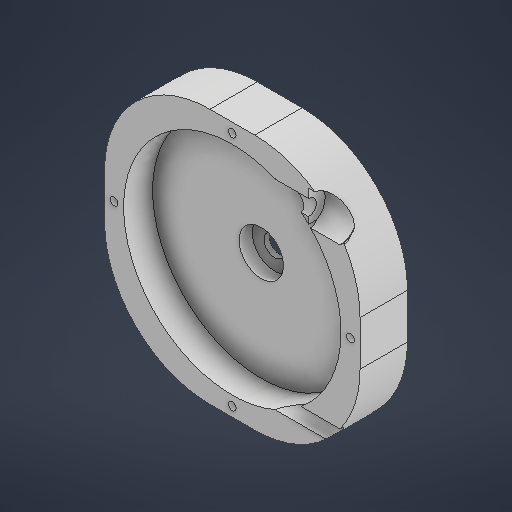
# Autodesk Inventor part: Case
Saved by Autodesk Inventor 2025.3 (Build 293356030, 356C)
## iProperties
Created: 2025-10-02
Part Number: Case
Material: Generic
Document SubType Name: Modeling
Designer: yo
Density: 1 g/cm^3
Appearance: Default
Author: yo
Autodesk Inventor part; units mm, degrees
ref_plane "YZ Plane" through (0, 0, 0) normal (1, 0, 0) x (0, 1, 0)
ref_plane "XZ Plane" through (0, 0, 0) normal (0, 1, 0) x (-1, 0, 0)
ref_plane "XY Plane" through (0, 0, 0) normal (0, 0, 1) x (1, 0, 0)
sketch "Sketch1" plane through (0, 0, 0) normal (0, 0, 1) x (1, 0, 0)
  line L0 (-8.5, 48.5) -> (8.5, 48.5)
  line L1 (48.5, 8.5) -> (48.5, -8.5)
  line L2 (8.5, -48.5) -> (-8.5, -48.5)
  line L3 (-48.5, -8.5) -> (-48.5, 8.5)
  circle A0 centre (0, 0) radius 41.25
  circle A1 centre (0, 0) radius 8.45
  circle A2 centre (0, 0) radius 4
  arc A3 (48.5, 8.5) -> (8.5, 48.5) centre (8.5, 8.5) ccw
  arc A4 (8.5, -48.5) -> (48.5, -8.5) centre (8.5, -8.5) ccw
  arc A5 (-48.5, -8.5) -> (-8.5, -48.5) centre (-8.5, -8.5) ccw
  arc A6 (-8.5, 48.5) -> (-48.5, 8.5) centre (-8.5, 8.5) ccw
  point P0 (-48.5, 48.5)
  point P1 (48.5, -48.5)
  point P2 (48.5, 48.5)
  point P3 (-48.5, -48.5)
  point P4 (0, 48.5)
  point P5 (48.5, 0)
  dimension "d0" = 97
  dimension "d1" = 82.5
  dimension "d2" = 16.9
  dimension "d3" = 8
  dimension "d10" = 40
  constraints: 8 end point, 8 point on circle, 8 point on line, 8 tangent, 7 centre point, 3 coincident, 3 equal radius, 2 midpoint, 2 parallel, 2 perpendicular, 1 horizontal, 1 horizontal alignment, 1 vertical alignment
  measures "d0" distance of point (-48.5, 48.5) point (48.5, 48.5)
  measures "d1" diameter of A0
  measures "d2" diameter of A1
  measures "d3" diameter of A2
  measures "d10" radius of A3
extrude "Extrusion1" add sketch "Sketch1" along normal blind 2 contours A1
extrude "Extrusion2" add sketch "Sketch1" along normal blind 7 contours A0
extrude "Extrusion3" add sketch "Sketch1" along normal blind 18 contours L0 A3 L1 A4 L2 A5 L3 A6
sketch "Sketch3" plane through (0, 0, 18) normal (0, 0, 1) x (1, 0, 0)
  circle A0 centre (0, 0) radius 41.25
  line L0 (21.9501, 34.925) -> (64.9501, 34.925)
  line L1 (41.9501, 40.25) -> (47.9501, 40.25)
  line L2 (49.9501, 42.25) -> (64.9501, 42.25)
  line L3 (40.9501, 41.25) -> (28.9501, 41.25)
  line L4 (49.9501, 42.25) -> (47.9501, 40.25)
  line L5 (40.9501, 41.25) -> (41.9501, 40.25)
  line L6 (47.9501, 40.25) -> (64.9501, 40.25) construction
  line L7 (41.9501, 40.25) -> (28.9501, 40.25) construction
  line L8 (64.9501, 42.25) -> (64.9501, 34.925)
  line L9 (28.9501, 37.925) -> (21.9501, 37.925)
  line L10 (28.9501, 37.925) -> (28.9501, 41.25)
  line L11 (21.9501, 37.925) -> (21.9501, 34.925) construction
  line L12 (21.9501, 34.925) -> (16.225193, 34.925)
  line L13 (21.9501, 37.925) -> (16.225193, 37.925)
  line L14 (16.225193, 34.925) -> (16.225193, 37.925)
  circle A1 centre (0, 0) radius 4
  line L15 (0, 0) -> (48.5, 0)
  line L16 (48.5, -8.5) -> (48.5, 8.5)
  line L17 (21.9501, -34.925) -> (64.9501, -34.925)
  line L18 (41.9501, -40.25) -> (47.9501, -40.25)
  line L19 (49.9501, -42.25) -> (64.9501, -42.25)
  line L20 (40.9501, -41.25) -> (28.9501, -41.25)
  line L21 (49.9501, -42.25) -> (47.9501, -40.25)
  line L22 (40.9501, -41.25) -> (41.9501, -40.25)
  line L23 (47.9501, -40.25) -> (64.9501, -40.25) construction
  line L24 (41.9501, -40.25) -> (28.9501, -40.25) construction
  line L25 (64.9501, -42.25) -> (64.9501, -34.925)
  line L26 (28.9501, -37.925) -> (21.9501, -37.925)
  line L27 (28.9501, -37.925) -> (28.9501, -41.25)
  line L28 (21.9501, -37.925) -> (21.9501, -34.925) construction
  line L29 (21.9501, -34.925) -> (16.225193, -34.925)
  line L30 (21.9501, -37.925) -> (16.225193, -37.925)
  line L31 (16.225193, -34.925) -> (16.225193, -37.925)
  line L32 (28.9501, -37.925) -> (64.9501, -37.925)
  point P0 (16.225193, -37.925)
  dimension "d12" = 10.65
  dimension "d13" = 14.65
  dimension "d14" = 12.65
  dimension "d15" = 45
  dimension "d16" = 45
  dimension "d17" = 15
  dimension "d18" = 6
  dimension "d19" = 12
  dimension "d21" = 7
  dimension "d22" = 6
  constraints: 64 end point, 14 symmetric about line, 9 horizontal, 4 vertical, 4 vertical alignment, 2 point on circle, 1 midpoint, 1 perpendicular, 1 point on line, 1 tangent
  measures "d12" diameter of L1 L0
  measures "d13" diameter of L2 L0
  measures "d14" diameter of L3 L0
  measures "d15" angle of L6 L4
  measures "d16" angle of L5 L7
  measures "d17" distance of L2.start L2.end
  measures "d18" distance of L1.start L1.end
  measures "d19" distance of L3.start L3.end
  measures "d21" distance of L9.start L9.end
  measures "d22" diameter of L9 L0
sketch "Sketch3 outline for Revolution1" plane through (0, 0, 18) normal (0, 0, 1) x (1, 0, 0)
  line L0 (64.9501, 34.925) -> (64.9501, 42.25)
  line L1 (21.9501, 34.925) -> (64.9501, 34.925)
  arc A0 (16.225193, 37.925) -> (21.9501, 34.925) centre (0, 0) cw
  line L2 (21.9501, 37.925) -> (16.225193, 37.925)
  line L3 (28.9501, 37.925) -> (21.9501, 37.925)
  line L4 (28.9501, 41.25) -> (28.9501, 37.925)
  line L5 (40.9501, 41.25) -> (28.9501, 41.25)
  line L6 (41.9501, 40.25) -> (40.9501, 41.25)
  line L7 (47.9501, 40.25) -> (41.9501, 40.25)
  line L8 (49.9501, 42.25) -> (47.9501, 40.25)
  line L9 (64.9501, 42.25) -> (49.9501, 42.25)
revolve "Revolution1" cut sketch "Sketch3 outline for Revolution1" angle 360 about axis through (21.9501, 34.925, 18) along (1, 0, 0)
sketch "Sketch3 outline for Revolution2" plane through (0, 0, 18) normal (0, 0, 1) x (1, 0, 0)
  line L0 (21.9501, -37.925) -> (28.9501, -37.925)
  line L1 (16.225193, -37.925) -> (21.9501, -37.925)
  arc A0 (21.9501, -34.925) -> (16.225193, -37.925) centre (0, 0) cw
  line L2 (64.9501, -34.925) -> (21.9501, -34.925)
  line L3 (64.9501, -37.925) -> (64.9501, -34.925)
  line L4 (28.9501, -37.925) -> (64.9501, -37.925)
revolve "Revolution2" cut sketch "Sketch3 outline for Revolution2" angle 360 about axis through (21.9501, -34.925, 18) along (1, 0, 0)
sketch "Sketch4" plane through (0, 0, 18) normal (0, 0, 1) x (1, 0, 0)
  line L0 (35.59556, -37.925) -> (16.225193, -37.925) construction
  arc A0 (16.225193, 37.925) -> (16.225193, -37.925) centre (0, 0) ccw construction
  line L1 (16.225193, 37.925) -> (28.9501, 37.925) construction
  line L2 (28.9501, 37.925) -> (28.9501, 41.25) construction
  line L3 (28.9501, 41.25) -> (31.466007, 41.25) construction
  arc A1 (31.466007, 41.25) -> (8.5, 48.5) centre (8.5, 8.5) ccw construction
  line L4 (8.5, 48.5) -> (-8.5, 48.5) construction
  arc A2 (-8.5, 48.5) -> (-48.5, 8.5) centre (-8.5, 8.5) ccw construction
  line L5 (-48.5, 8.5) -> (-48.5, -8.5) construction
  arc A3 (-48.5, -8.5) -> (-8.5, -48.5) centre (-8.5, -8.5) ccw construction
  line L6 (-8.5, -48.5) -> (8.5, -48.5) construction
  arc A4 (8.5, -48.5) -> (35.59556, -37.925) centre (8.5, -8.5) ccw construction
  line L7 (26.121962, -31.925) -> (40.923284, -31.925) construction
  arc A5 (40.923284, -31.925) -> (48.5, -8.5) centre (8.5, -8.5) ccw construction
  line L8 (48.5, -8.5) -> (48.5, 8.5) construction
  arc A6 (48.5, 8.5) -> (42.482201, 29.6) centre (8.5, 8.5) ccw construction
  line L9 (42.482201, 29.6) -> (41.9501, 29.6) construction
  line L10 (41.9501, 29.6) -> (40.9501, 28.6) construction
  line L11 (40.9501, 28.6) -> (29.725452, 28.6) construction
  arc A7 (26.121962, -31.925) -> (29.725452, 28.6) centre (0, 0) ccw construction
  line L12 (-48.5, 0) -> (-41.25, 0) construction
  circle A8 centre (-44.875, 0) radius 1.485
  circle A9 centre (0, -44.875) radius 1.485
  circle A10 centre (44.875, 0) radius 1.485
  circle A11 centre (0, 44.875) radius 1.485
  dimension "d25" = 2.97
  dimension "d28" = 360
  constraints: 4 centre point, 2 end point, 2 midpoint, 1 point on circle, 9 other
  measures "d25" diameter of A8
extrude "Extrusion4" cut sketch "Sketch4" against normal through all
body "Solid1"
